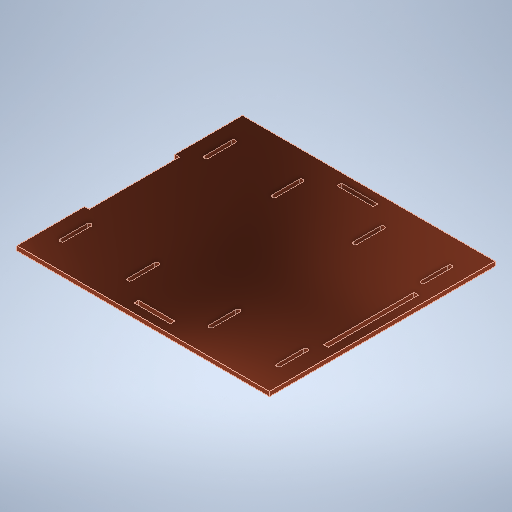
# Autodesk Inventor part: base_2
Saved by Autodesk Inventor 2025.3 (Build 293356030, 356C)
## iProperties
Created: 2026-06-26
Part Number: base_2
Material: Generic
Document SubType Name: Modeling
Designer: user
Density: 1 g/cm^3
Appearance: Copper - Polished
Author: user
Autodesk Inventor part; units mm, degrees
ref_plane "YZ Plane" through (0, 0, 0) normal (1, 0, 0) x (0, 1, 0)
ref_plane "XZ Plane" through (0, 0, 0) normal (0, 1, 0) x (-1, 0, 0)
ref_plane "XY Plane" through (0, 0, 0) normal (0, 0, 1) x (1, 0, 0)
sketch "Sketch1" plane through (0, 0, 0) normal (0, 1, 0) x (-1, 0, 0)
  line L0 (0, 0) -> (-280, 0)
  line L1 (-280, 0) -> (-280, -250)
  line L2 (-280, -250) -> (0, -250)
  line L3 (0, -250) -> (0, 0)
  line L4 (0, -125) -> (-280, -125) construction
  line L5 (-140, 0) -> (-140, -250) construction
  line L6 (-57.5, 0) -> (-57.5, -250) construction
  line L7 (-203, 0) -> (-203, -250) construction
  line L8 (-20, -220) -> (-20, -190) construction
  line L9 (-20, -220) -> (-20, -190) construction
  line L10 (-17.75, -220) -> (-17.75, -190)
  line L11 (-22.25, -190) -> (-22.25, -220)
  arc A0 (-22.25, -220) -> (-17.75, -220) centre (-20, -220) ccw
  arc A1 (-17.75, -190) -> (-22.25, -190) centre (-20, -190) ccw
  line L12 (-95, -220) -> (-95, -190) construction
  line L13 (-95, -220) -> (-95, -190) construction
  line L14 (-97.25, -220) -> (-97.25, -190)
  line L15 (-92.75, -190) -> (-92.75, -220)
  arc A2 (-97.25, -220) -> (-92.75, -220) centre (-95, -220) ccw
  arc A3 (-92.75, -190) -> (-97.25, -190) centre (-95, -190) ccw
  line L16 (-160, -240) -> (-120, -240)
  line L17 (-120, -240) -> (-120, -235)
  line L18 (-120, -235) -> (-160, -235)
  line L19 (-160, -235) -> (-160, -240)
  line L20 (-260, -220) -> (-260, -190) construction
  line L21 (-260, -220) -> (-260, -190) construction
  line L22 (-262.25, -220) -> (-262.25, -190)
  line L23 (-257.75, -190) -> (-257.75, -220)
  arc A4 (-262.25, -220) -> (-257.75, -220) centre (-260, -220) ccw
  arc A5 (-257.75, -190) -> (-262.25, -190) centre (-260, -190) ccw
  line L24 (-187.25, -190) -> (-187.25, -220)
  line L25 (-185, -220) -> (-185, -190) construction
  line L26 (-182.75, -220) -> (-182.75, -190)
  arc A6 (-187.25, -220) -> (-182.75, -220) centre (-185, -220) ccw
  line L27 (-185, -220) -> (-185, -190) construction
  arc A7 (-182.75, -190) -> (-187.25, -190) centre (-185, -190) ccw
  line L28 (-140, -250) -> (-140, 0) construction
  line L29 (-20, -30) -> (-20, -60) construction
  line L30 (-20, -30) -> (-20, -60) construction
  line L31 (-17.75, -30) -> (-17.75, -60)
  line L32 (-22.25, -60) -> (-22.25, -30)
  arc A8 (-17.75, -30) -> (-22.25, -30) centre (-20, -30) ccw
  arc A9 (-22.25, -60) -> (-17.75, -60) centre (-20, -60) ccw
  line L33 (-92.75, -60) -> (-92.75, -30)
  line L34 (-95, -30) -> (-95, -60) construction
  line L35 (-97.25, -30) -> (-97.25, -60)
  arc A10 (-92.75, -30) -> (-97.25, -30) centre (-95, -30) ccw
  line L36 (-95, -30) -> (-95, -60) construction
  arc A11 (-97.25, -60) -> (-92.75, -60) centre (-95, -60) ccw
  line L37 (-160, -10) -> (-120, -10)
  line L38 (-120, -10) -> (-120, -15)
  line L39 (-120, -15) -> (-160, -15)
  line L40 (-160, -15) -> (-160, -10)
  arc A12 (-257.75, -30) -> (-262.25, -30) centre (-260, -30) ccw
  line L41 (-257.75, -60) -> (-257.75, -30)
  line L42 (-260, -30) -> (-260, -60) construction
  line L43 (-260, -30) -> (-260, -60) construction
  arc A13 (-262.25, -60) -> (-257.75, -60) centre (-260, -60) ccw
  line L44 (-262.25, -30) -> (-262.25, -60)
  line L45 (-187.25, -60) -> (-187.25, -30)
  line L46 (-185, -30) -> (-185, -60) construction
  line L47 (-185, -30) -> (-185, -60) construction
  arc A14 (-187.25, -60) -> (-182.75, -60) centre (-185, -60) ccw
  line L48 (-182.75, -30) -> (-182.75, -60)
  arc A15 (-182.75, -30) -> (-187.25, -30) centre (-185, -30) ccw
  line L49 (-270, -102.5) -> (-270, -152.5)
  line L50 (-270, -152.5) -> (-270, -175)
  line L51 (-270, -175) -> (-265, -175)
  line L52 (-265, -175) -> (-265, -75)
  line L53 (-265, -75) -> (-270, -75)
  line L54 (-270, -75) -> (-270, -102.5)
  line L55 (0, -75) -> (-5, -75)
  line L56 (-5, -75) -> (-5, -175)
  line L57 (-5, -175) -> (0, -175)
  line L58 (0, -175) -> (0, -75)
  point P0 (-20, -205)
  point P1 (-95, -205)
  point P2 (-260, -205)
  point P3 (-185, -205)
  point P4 (-20, -45)
  point P5 (-95, -45)
  point P6 (-260, -45)
  point P7 (-185, -45)
  point P8 (0, -175)
  point P9 (-95, -205)
  point P10 (-20, -205)
  dimension "d2" = 30
  dimension "d4" = 30
  dimension "d6" = 2.25
  dimension "d9" = 40
  dimension "d13" = 10
  dimension "d14" = 5
  dimension "d16" = 20
  dimension "d21" = 5
  dimension "d22" = 5
  dimension "d26" = 50
  dimension "d27" = 50
  dimension "d28" = 10
  dimension "d30" = 250
  dimension "d31" = 280
  dimension "d32" = 75
  dimension "d33" = 20
  dimension "d34" = 100
  dimension "d35" = 75
  constraints: 134 end point, 55 symmetric about line, 32 point on circle, 16 centre point, 8 equal length, 7 midpoint, 6 point on line, 5 perpendicular, 4 tangent, 3 horizontal, 1 vertical, 14 other
  measures "d2" distance of L8.start L8.end
  measures "d4" distance from line of L2 L8.start
  measures "d6" radius of A0
  measures "d9" distance of L18.end L17.end
  measures "d13" distance between parallel lines of L2 L16
  measures "d14" distance between parallel lines of L18 L16
  measures "d16" distance between parallel lines of L5 L19
  measures "d21" distance of L57.end L56.end
  measures "d22" distance between parallel lines of L50 L52
  measures "d26" distance between parallel lines of L4 L53
  measures "d27" distance between parallel lines of L4 L51
  measures "d28" distance between parallel lines of L1 L49
  measures "d30" distance between parallel lines of L0 L2
  measures "d31" distance between parallel lines of L3 L1
  measures "d32" distance of point (-95, -205) point (-20, -205)
  measures "d33" distance from line of L3 point (-20, -205)
  measures "d34" distance between parallel lines of L57 L55
  measures "d35" distance between parallel lines of L2 L57
extrude "Extrusion1" add sketch "Sketch1" along normal blind 5 contours L3 L55 L56 L57 L2 L1 L0
body "Solid1"
